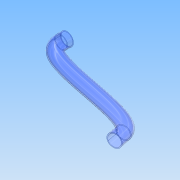
# Autodesk Inventor part: Top_End Pipe 4
Saved by Autodesk Inventor 2018.1 (Build 221171000, 171)
## iProperties
Created: 2019-03-22
Part Number: Top_End Pipe 4
Material: PMMA Plastic
Document SubType Name: Modeling
Designer: James
Density: 1.188 g/cm^3
Appearance: Clear - Blue
Author: James
Autodesk Inventor part; units mm, degrees
ref_plane "YZ Plane" through (0, 0, 0) normal (1, 0, 0) x (0, 1, 0)
ref_plane "XZ Plane" through (0, 0, 0) normal (0, 1, 0) x (-1, 0, 0)
ref_plane "XY Plane" through (0, 0, 0) normal (0, 0, 1) x (1, 0, 0)
sketch "Sketch1" plane through (0, 0, 0) normal (0, 1, 0) x (-1, 0, 0)
  circle A0 centre (0, 0) radius 23
  circle A1 centre (0, 0) radius 20
  dimension "d0" = 46
  dimension "d1" = 40
  constraints: 2 centre point, 2 coincident
  measures "d0" diameter of A0
  measures "d1" diameter of A1
sketch3d "3D Sketch1"
  spline S0 degree 4 poles (0, 0, 0) (0, -50, 0) (0, -50, -40) (325, -50, -40) (339.9526, -123.4944, -40) knots 1 1 1 1 1 2 2 2 2 2
  dimension "d2" = 50
  dimension "d5" = 78.5
  dimension "d6" = 75
  dimension "d13" = 40
  dimension "d14" = 325
sweep "Sweep1" add profiles "Sketch1" path "3D Sketch1"
sketch "Sketch2" plane through (0, 0, 0) normal (0, 1, 0) x (1, 0, 0)
  spline S0 degree 6 poles (-20, 0) (-20, 33.2309) (21.091, 38.0022) (54.9823, 0) (21.091, -38.0022) (-20, -33.2309) (-20, 0) knots 0 0 0 0 0 0 0 1 1 1 1 1 1 1 weights 1.669078 1.03673 1.038347 0.853534 1.038347 1.03673 1.669078 projected
  circle A0 centre (0, 0) radius 23 projected
  point P0 (-23, 0)
  constraints: 1 horizontal alignment, 1 other
extrude "Extrusion1" add sketch "Sketch2" along normal blind 20
sketch "Sketch4" plane through (339.9526, -123.4944, -40) normal (0.1993679, -0.9799247, 0) x (0.9799247, 0.1993679, 0)
  spline S0 degree 6 poles (-18.5435, -7.4925) (-6.0943, -38.3034) (33.7917, -27.3335) (50.9783, 20.5979) (5.3184, 43.136) (-30.9927, 23.3183) (-18.5435, -7.4925) knots 0 0 0 0 0 0 0 1 1 1 1 1 1 1 weights 1.669078 1.03673 1.038347 0.853534 1.038347 1.03673 1.669078 projected
  circle A0 centre (0, 0) radius 23 projected
  point P0 (-308.5071, 40)
  point P1 (-21.195, -8.9315)
  constraints: 2 other
extrude "Extrusion2" add sketch "Sketch4" along normal blind 40 contours S0 picked at (-0.7735, 21.8432)
body "Solid1"
